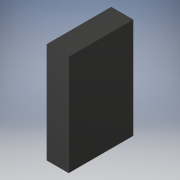
# Autodesk Inventor part: Stepperdriver
Saved by Autodesk Inventor 2019 (Build 230136000, 136)
## iProperties
Created: 2021-11-05
Part Number: Stepperdriver
Material: Generisch
Document SubType Name: Modeling
Designer: Bergi
Density: 1 g/cm^3
Appearance: Glatt - Schwarz
Author: Bergi
Autodesk Inventor part; units mm, degrees
ref_plane "YZ Plane" through (0, 0, 0) normal (1, 0, 0) x (0, 1, 0)
ref_plane "XZ Plane" through (0, 0, 0) normal (0, 1, 0) x (-1, 0, 0)
ref_plane "XY Plane" through (0, 0, 0) normal (0, 0, 1) x (1, 0, 0)
sketch "Skizze1" plane through (0, 0, 0) normal (0, 0, 1) x (1, 0, 0)
  line L0 (-12.75, -59) -> (12.75, -59)
  line L1 (12.75, -59) -> (12.75, 59)
  line L2 (12.75, 59) -> (-12.75, 59)
  line L3 (-12.75, 59) -> (-12.75, -59)
  line L4 (-12.75, -59) -> (12.75, 59) construction
  line L5 (12.75, -59) -> (-12.75, 59) construction
  point P0 (0, 0)
  dimension "d0" = 25.5
  dimension "d1" = 118
  constraints: 12 end point, 2 midpoint, 2 parallel, 1 horizontal, 1 perpendicular
  measures "d0" distance of L2.end L1.end
  measures "d1" distance of L1.end L0.end
extrude "Extrusion1" add sketch "Skizze1" along normal blind 75.5
